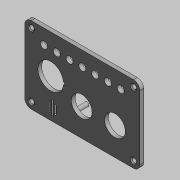
# Autodesk Inventor part: Пластина для дальномера
Saved by Autodesk Inventor 2017 (Build 210142000, 142)
## iProperties
Part Number: Пластина для дальномера
Material: Типовой
Document SubType Name: Обычные детали
Designer: root
Appearance: Типовой
Author: root
Autodesk Inventor part; units mm, degrees
ref_plane "Плоскость YZ" through (0, 0, 0) normal (1, 0, 0) x (0, 1, 0)
ref_plane "Плоскость XZ" through (0, 0, 0) normal (0, 1, 0) x (-1, 0, 0)
ref_plane "Плоскость XY" through (0, 0, 0) normal (0, 0, 1) x (1, 0, 0)
sketch "Эскиз1" plane through (0, 0, 0) normal (0, 0, 1) x (1, 0, 0)
  line L0 (-40, -30) -> (40, -30)
  line L1 (45, -25) -> (45, 25)
  line L2 (40, 30) -> (-40, 30)
  line L3 (-45, 25) -> (-45, -25)
  line L4 (-45, -30) -> (45, 30) construction
  line L5 (45, -30) -> (-45, 30) construction
  circle A0 centre (-20, 18.4812) radius 2.75
  circle A1 centre (20, 18.4812) radius 2.75
  circle A2 centre (0, 18.4812) radius 2.75
  circle A3 centre (10, 18.4812) radius 2.75
  circle A4 centre (30, 18.4812) radius 2.75
  circle A5 centre (-10, 18.4812) radius 2.75
  circle A6 centre (-30, 18.4812) radius 2.75
  arc A7 (-40, 30) -> (-45, 25) centre (-40, 25) ccw
  arc A8 (45, 25) -> (40, 30) centre (40, 25) ccw
  arc A9 (40, -30) -> (45, -25) centre (40, -25) ccw
  arc A10 (-45, -25) -> (-40, -30) centre (-40, -25) ccw
  circle A11 centre (-0.508, -8.2758) radius 8.1
  circle A12 centre (25.492, -8.2758) radius 8.1
  line L6 (-14.7884, -1) -> (-13.8217, -1)
  line L7 (-13.8217, -1) -> (-13.8217, 1)
  line L8 (-13.8217, 1) -> (-14.7884, 1)
  line L9 (-15.8217, -1) -> (-13.8217, 1) construction
  line L10 (-13.8217, -1) -> (-15.8217, 1) construction
  arc A13 (-14.7884, 1) -> (-14.7884, -1) centre (-24.7383, 0) ccw
  point P0 (0, 0)
  point P1 (7.592, -8.2758)
  point P2 (-14.8217, 0)
  dimension "d12" = 16.2
  dimension "d0" = 90
  dimension "d1" = 60
  dimension "d5" = 5.5
  dimension "d6" = 5.5
  dimension "d7" = 5.5
  dimension "d8" = 5.5
  dimension "d9" = 5.5
  dimension "d10" = 5
  dimension "d13" = 16.2
  dimension "d56" = 26
  dimension "d72" = 2
  dimension "d73" = 2
  constraints: 22 end point, 13 centre point, 10 point on circle, 8 point on line, 8 tangent, 4 midpoint, 3 equal radius, 3 parallel, 2 horizontal, 2 perpendicular, 1 horizontal alignment, 2 other
  measures "d0" distance of L5.end L4.end
  measures "d1" distance of L4.end L5.start
  measures "d5" diameter of A0
  measures "d6" diameter of A1
  measures "d7" diameter of A2
  measures "d8" diameter of A3
  measures "d9" diameter of A4
  measures "d10" radius of A7
  measures "d13" diameter of A12
  measures "d56" distance of point (-0.508, -8.276) A12.centre
  measures "d72" distance of L10.end L7.end
  measures "d73" distance of L7.end L6.end
extrude "Выдавливание1" add sketch "Эскиз1" along normal blind 3
sketch "Эскиз5" plane through (0, 0, 0) normal (0, 0, -1) x (-1, 0, 0)
  circle A0 centre (23.2586, -20.8667) radius 6 construction
  line L0 (23.2586, -26.8667) -> (23.2586, -14.8667) construction
  line L1 (22.7526, -26.3606) -> (22.7526, -15.3728)
  line L2 (23.7647, -15.3728) -> (23.7647, -26.3606)
  arc A1 (22.7526, -26.3606) -> (23.7647, -26.3606) centre (23.2586, -26.3606) ccw
  arc A2 (23.7647, -15.3728) -> (22.7526, -15.3728) centre (23.2586, -15.3728) ccw
  line L3 (25.4054, -17.1002) -> (25.4054, -24.6332) construction
  line L4 (25.976, -17.6708) -> (25.976, -24.0626)
  line L5 (24.8347, -24.0626) -> (24.8347, -17.6708)
  arc A3 (25.976, -17.6708) -> (24.8347, -17.6708) centre (25.4054, -17.6708) ccw
  arc A4 (24.8347, -24.0626) -> (25.976, -24.0626) centre (25.4054, -24.0626) ccw
  line L6 (21.1119, -17.1002) -> (21.1119, -24.6332) construction
  line L7 (20.5412, -17.6708) -> (20.5412, -24.0626)
  line L8 (21.6825, -24.0626) -> (21.6825, -17.6708)
  arc A5 (21.6825, -17.6708) -> (20.5412, -17.6708) centre (21.1119, -17.6708) ccw
  arc A6 (20.5412, -24.0626) -> (21.6825, -24.0626) centre (21.1119, -24.0626) ccw
  point P0 (0, 0)
  point P1 (21.1119, -20.8667)
  dimension "d42" = 12
  constraints: 24 end point, 20 point on circle, 8 tangent, 7 centre point, 6 point on line, 2 parallel
  measures "d42" diameter of A0
extrude "Выдавливание3" cut sketch "Эскиз5" against normal blind 11
sketch "Эскиз7" plane through (0, 0, 0) normal (0, 0, -1) x (-1, 0, 0)
  line L0 (22.7526, -26.3606) -> (22.7526, -15.3728) projected
  line L1 (23.7647, -15.3728) -> (23.7647, -26.3606) projected
  arc A0 (23.7647, -15.3728) -> (22.7526, -15.3728) centre (23.2586, -15.3728) ccw projected
  circle A1 centre (23.2586, -20.8667) radius 6.1
  circle A2 centre (23.2586, -20.8667) radius 7.15
  point P0 (0, 0)
  dimension "d50" = 12.2
  dimension "d51" = 14.3
  constraints: 2 centre point, 1 coincident
  measures "d50" diameter of A1
  measures "d51" diameter of A2
extrude "Выдавливание5" add sketch "Эскиз7" along normal blind 5
sketch "Эскиз8" plane through (0, 0, 0) normal (0, 0, -1) x (-1, 0, 0)
  circle A0 centre (-25.492, -8.2758) radius 8.1 projected
  circle A1 centre (0.508, -8.2758) radius 8.1 projected
  line L0 (-33.492, -16.7758) -> (8.508, 0.2242) construction
  line L1 (8.508, -16.7758) -> (-33.492, 0.2242) construction
  circle A2 centre (-33.492, 0.2242) radius 1.75
  circle A3 centre (-33.492, -16.7758) radius 1.75
  circle A4 centre (8.508, 0.2242) radius 1.75
  circle A5 centre (8.508, -16.7758) radius 1.75
  point P0 (0, 0)
  dimension "d57" = 42
  dimension "d58" = 17
  dimension "d59" = 3.5
  dimension "d60" = 3.5
  dimension "d61" = 3.5
  dimension "d62" = 3.5
  constraints: 4 centre point, 4 coincident, 4 end point
  measures "d57" distance of L1.end L0.end
  measures "d58" distance of L0.end L1.start
  measures "d59" diameter of A2
  measures "d60" diameter of A3
  measures "d61" diameter of A4
  measures "d62" diameter of A5
extrude "Выдавливание6" add sketch "Эскиз8" along normal blind 9 contours A2 | A3 | A4 | A5
sketch "Эскиз9" plane through (33.492, 0.2242, -9) normal (0, 0, -1) x (-1, 0, 0)
  circle A0 centre (0, 0) radius 1.75 projected
  circle A1 centre (42, 0) radius 1.75 projected
  circle A2 centre (42, -17) radius 1.75 projected
  circle A3 centre (0, -17) radius 1.75 projected
  point P0 (33.492, -0.2242)
  constraints: 4 coincident
hole "Отверстие3" at (33.492, 0.2242, -9) at (-8.508, 0.2242, -9) at (-8.508, -16.7758, -9) at (33.492, -16.7758, -9) direction (0, 0, 1) diameter 2 depth 5 tip angle 118
sketch "Эскиз10" plane through (0, 0, 3) normal (0, 0, 1) x (1, 0, 0)
  arc A0 (-40, 30) -> (-45, 25) centre (-40, 25) ccw projected
  circle A1 centre (-40, 25) radius 2.5
  circle A2 centre (40, 25) radius 2.5
  circle A3 centre (-40, -25) radius 2.5
  circle A4 centre (40, -25) radius 2.5
  point P0 (0, 0)
  dimension "d74" = 5
  dimension "d75" = 5
  dimension "d76" = 5
  dimension "d77" = 5
  constraints: 4 centre point, 1 coincident
  measures "d74" diameter of A1
  measures "d75" diameter of A2
  measures "d76" diameter of A3
  measures "d77" diameter of A4
hole "Отверстие4" at (-40, 25, 3) at (-40, -25, 3) at (40, -25, 3) at (40, 25, 3) direction (0, 0, -1) diameter 3.5 depth 5 tip angle 118 countersink diameter 5 countersink angle 90
